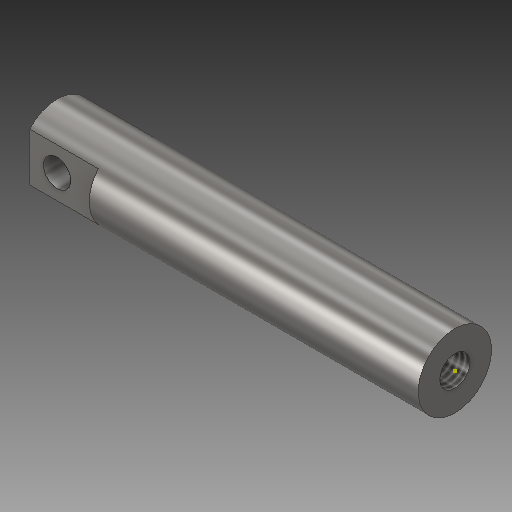
# Autodesk Inventor part: Part3
Saved by Autodesk Inventor 2019 (Build 230136000, 136)
## iProperties
Created: 2018-10-25
Part Number: Part3
Material: Steel
Document SubType Name: Modeling
Designer: Isaac
Density: 7.85 g/cm^3
Appearance: Semi-Polished
Author: Isaac
Autodesk Inventor part; units mm, degrees
ref_plane "YZ Plane" through (0, 0, 0) normal (1, 0, 0) x (0, 1, 0)
ref_plane "XZ Plane" through (0, 0, 0) normal (0, 1, 0) x (-1, 0, 0)
sketch "Sketch1" plane through (0, 0, 0) normal (1, 0, 0) x (0, 1, 0)
  circle A0 centre (0, 0) radius 8
  dimension "d0" = 16
  constraints: 1 centre point, 1 coincident
  measures "d0" diameter of A0
extrude "Extrusion1" add sketch "Sketch1" against normal blind 87
ref_plane "Work Plane1" through (0, 0, 0) normal (0, 0, 1) x (-1, 0, 0)
sketch "Sketch2" plane through (0, 0, 0) normal (0, 0, 1) x (1, 0, 0)
  point P0 (0, 0)
ref_plane "Work Plane2" through (0, 0, -6) normal (0, 0, 1) x (-1, 0, 0)
sketch "Sketch3" plane through (0, 0, -6) normal (0, 0, 1) x (-1, 0, 0)
  line L0 (72, -14.6866) -> (87, -14.6866)
  line L1 (87, -14.6866) -> (87, 13.5616)
  line L2 (87, 13.5616) -> (72, 13.5616)
  line L3 (72, 13.5616) -> (72, -14.6866)
  line L4 (87, -8) -> (87, 8) projected
  point P0 (0, 0)
  dimension "d5" = 15
  dimension "d6" = 0
  constraints: 8 end point, 2 parallel, 1 horizontal, 1 perpendicular
  measures "d5" distance of L0.start L0.end
  measures "d6" distance between parallel lines of L4 L1
extrude "Extrusion2" cut sketch "Sketch3" against normal blind 87
mirror "Mirror1" about plane through (0, 0, 0) normal (0, 0, 1) of "Extrusion2"
sketch "Sketch4" plane through (0, 0, 0) normal (0, 0, 1) x (-1, 0, 0)
  circle A0 centre (81, 0) radius 3
  line L0 (87, -5.2915) -> (87, 5.2915) projected
  point P0 (0, 0)
  dimension "d9" = 6
  dimension "d10" = 6
  constraints: 1 centre point
  measures "d9" distance from line of A0.centre L0
  measures "d10" diameter of A0
extrude "Extrusion3" cut sketch "Sketch4" along normal mid plane 20
hole "Hole1" at (0, 0, 0) direction (-1, 0, 0) diameter 6.647 depth 50 tip angle 118 thread size "M8x1.25" class "6H" standard "ISO Metric profile"
body "Solid1"
